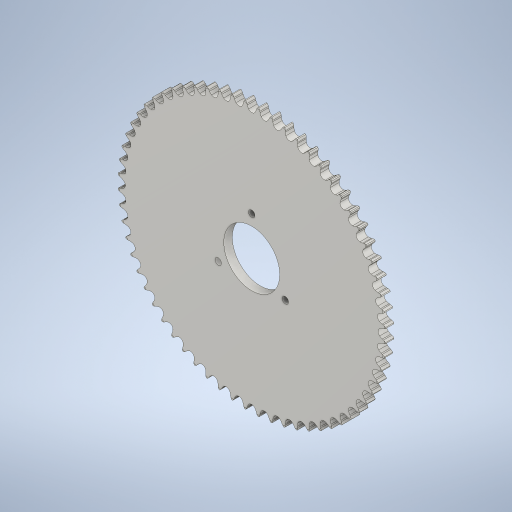
# Autodesk Inventor part: Roller Chain Sprocket2
Saved by Autodesk Inventor 2023 (Build 270158000, 158)
## iProperties
CustomPartVersion: 1
Created: 2023-09-03
Part Number: Roller Chain Sprocket2
Material: Steel
Document SubType Name: Modeling
Designer: sigit
Density: 1 g/cm^3
Appearance: Steel
Author: sigit
Autodesk Inventor part; units mm, degrees
ref_plane "YZ Plane" through (0, 0, 0) normal (1, 0, 0) x (0, 1, 0)
ref_plane "XZ Plane" through (0, 0, 0) normal (0, 1, 0) x (-1, 0, 0)
sketch "Theoretical Tooth Profile" plane through (0, 0, 0) normal (0, 0, 1) x (1, 0, 0)
  circle A0 centre (0, 0) radius 81.5201 construction
  line L0 (0, 0) -> (0, 81.5201) construction
  line L1 (0, 0) -> (7.9904, 81.1275) construction
  circle A1 centre (0, 0) radius 83.8219
  arc A2 (-1.9503, 80.1063) -> (1.9503, 80.1063) centre (0, 81.5201) ccw
  line L2 (0, 81.5201) -> (7.9904, 81.1275) construction
  line L3 (0, 81.5201) -> (3.0897, 83.7597) construction
  line L4 (3.0897, 83.7597) -> (-2.8027, 81.7523) construction
  arc A3 (3.7916, 83.7361) -> (3.0339, 82.4311) centre (6.67, 81.1924) ccw
  arc A4 (-3.0339, 82.4311) -> (-3.7916, 83.7361) centre (-6.67, 81.1924) ccw
  line L5 (-6.67, 81.1924) -> (-3.0339, 82.4311) construction
  arc A5 (-2.8027, 81.7523) -> (-1.9503, 80.1063) centre (3.0897, 83.7597) ccw
  line L6 (-2.8027, 81.7523) -> (-3.0339, 82.4311)
  arc A6 (1.9503, 80.1063) -> (2.8027, 81.7523) centre (-3.0897, 83.7597) ccw
  line L7 (3.0339, 82.4311) -> (2.8027, 81.7523)
  line L8 (0, 0) -> (4.1129, 83.7209) construction
  point P0 (3.9952, 81.3238)
  dimension "d0" = 163.0401
  dimension "d2" = 5.625
  dimension "d3" = 2.4089
  dimension "d10" = 125.938
  dimension "d11" = 17.125
  dimension "d12" = 3.816
  dimension "d13" = 6.2248
  dimension "d14" = 6.678
  dimension "d23" = 2.4
  constraints: 18 end point, 15 point on circle, 7 centre point, 3 coincident, 3 point on line, 3 symmetric about line, 3 tangent, 1 equal radius, 1 midpoint, 1 parallel, 1 vertical, 1 other
  measures "d0" diameter of A0
  measures "d2" angle of L1 L0
  measures "d3" radius of A2
  measures "d10" angle of L3 L0
  measures "d11" angle of L4 L3
  measures "d12" distance of L2.start L3.end
  measures "d13" distance of L3.end L4.end
  measures "d14" distance of A3.centre L0.end
  measures "d23" distance from line of L8.end L2
sketch "Tooth Profile" plane through (0, 0, 0) normal (0, 0, 1) x (1, 0, 0)
  arc A0 (-2.2533, 80.6685) -> (2.2533, 80.6685) centre (0, 81.5201) ccw
  arc A1 (3.5749, 83.7456) -> (2.2533, 80.6685) centre (37.5921, 67.3128) ccw
  arc A2 (-2.2533, 80.6685) -> (-3.5749, 83.7456) centre (-37.5921, 67.3128) ccw
  line L0 (0, 0) -> (0, 81.5201) construction
  line L1 (0, 81.5201) -> (2.2533, 80.6685) construction
  line L2 (0, 81.5201) -> (-2.2533, 80.6685) construction
  circle A3 centre (0, 0) radius 83.8219 projected
  dimension "d44" = 138.594
  dimension "d45" = 37.7784
  dimension "d46" = 2.4089
  constraints: 9 point on circle, 6 end point, 3 centre point, 2 tangent, 1 coincident, 1 equal radius, 1 vertical, 1 other
  measures "d44" angle of L2 L1
  measures "d45" radius of A1
  measures "d46" radius of A0
sketch "Section Profile" plane through (0, 0, 0) normal (1, 0, 0) x (0, 1, 0)
  line L0 (83.8219, 0) -> (-83.8219, 0) projected
  line L1 (73.3499, 2.6598) -> (-73.3499, 2.6598)
  line L2 (-73.3499, 2.6598) -> (-73.3499, -2.6598)
  line L3 (-73.3499, -2.6598) -> (73.3499, -2.6598)
  line L4 (73.3499, -2.6598) -> (73.3499, 2.6598)
  line L5 (73.3499, 2.6598) -> (83.8219, 2.6598) construction
  line L6 (83.8219, 2.6598) -> (83.8219, -2.6598) construction
  line L7 (83.8219, -2.6598) -> (73.3499, -2.6598) construction
  line L8 (73.3499, -2.6598) -> (73.3499, 2.6598)
  arc A0 (83.8219, 2.6118) -> (82.9468, 2.6598) centre (82.9468, -5.3402) ccw
  arc A1 (82.9468, -2.6598) -> (83.8219, -2.6118) centre (82.9468, 5.3402) ccw
  line L9 (82.9468, 2.6598) -> (0, 2.6598)
  line L10 (0, 2.6598) -> (0, -2.6598)
  line L11 (0, -2.6598) -> (82.9468, -2.6598)
  line L12 (0, 2.6598) -> (0, -2.6598)
  line L13 (83.8219, 2.6118) -> (83.8219, -2.6118)
  point P0 (0, 0)
  point P1 (0, 0)
  dimension "d30" = 5.3196
  dimension "d31" = 146.6997
  dimension "d32" = 5.3196
  dimension "d33" = 0.048
  dimension "d34" = 8
  dimension "d43" = 2.6598
  constraints: 26 end point, 7 midpoint, 5 perpendicular, 4 parallel, 4 point on circle, 3 point on line, 3 symmetric about line, 2 centre point, 2 horizontal, 2 tangent, 1 collinear, 1 other
  measures "d30" distance between parallel lines of L7 L5
  measures "d31" distance between parallel lines of L2 L4
  measures "d32" distance between parallel lines of L3 L1
  measures "d33" distance from line of L13.start L5
  measures "d34" radius of A0
  measures "d43" distance between parallel lines of L3 L0
revolve "Shroud" add sketch "Section Profile" angle 360 about axis through (0, 0, 2.6598) along (0, 0, -1) contours L10 L3 L2 L0 | L0 L2 L1 L10
revolve "Strand" add sketch "Section Profile" angle 360 about axis through (0, 0, 2.6598) along (0, 0, -1) contours L13 A1 L11 L4 L0 | L0 L4 L9 A0 L13 | L4 L3 L10 L0 | L0 L10 L1 L4
pattern_of_one "Strand Pattern"
extrude "Theoretical Tooth" cut sketch "Theoretical Tooth Profile" along normal through all both and the other way through all contours A3 L7 A6 A2 A5 L6 A4 A1 picked at (0.4214, 81.3417)
extrude "Tooth" [suppressed]
pattern_circular "Tooth Pattern" count 64 over 360 about axis through (0, 0, -10) along (0, 0, 1) of "Theoretical Tooth"
ref_plane "Timing Plane" through (0, 81.5201, 0) normal (1, 0, 0) x (0, 1, 0)
sketch "Sketch4" plane through (0, 81.5201, 2.6598) normal (0, 0, 1) x (1, 0, 0)
  circle A0 centre (0, -81.5201) radius 17.5
  circle A1 centre (0, -57.2701) radius 2
  circle A2 centre (-21.0011, -93.6451) radius 2
  circle A3 centre (21.0011, -93.6451) radius 2
  circle A4 centre (0, -81.5201) radius 17.5
  dimension "d51" = 35
  dimension "d54" = 4
  dimension "d55" = 360
  dimension "d56" = 24.25
  dimension "d57" = 35
  constraints: 5 centre point, 2 coincident, 7 other
  measures "d51" diameter of A0
  measures "d54" diameter of A1
  measures "d56" distance of A1.centre point (0, -81.52)
  measures "d57" diameter of A4
extrude "Extrusion4" cut sketch "Sketch4" against normal through all
equation "\"d3\" = 0.5 * da_Dr + da_SC"
equation "\"d12\" = 0.8 * da_Dr"
equation "\"d13\" = 1.3 * da_Dr + da_SC"
equation "\"d14\" = 1.4 * da_Dr"
equation "\"d23\" = da_Ha"
equation "\"d44\" = da_Alfa"
equation "\"d45\" = da_Re"
equation "\"d46\" = da_Ri"
equation "\"d30\" = da_Bf"
equation "\"d31\" = da_Ds"
equation "\"d32\" = da_Bs"
equation "\"d33\" = da_Ba"
equation "\"d34\" = da_Rx"
equation "\"d40\" = da_pt"
equation "\"form_type\" = 0"
equation "\"da_p\" = 8"
equation "\"da_Dr\" = 4.77"
equation "\"da_SC\" = 0.02385"
equation "\"da_Ha\" = 2.4"
equation "\"da_pt\" = 11.6"
equation "\"da_Bf\" = 5.3196"
equation "\"da_Ba\" = 0.048"
equation "\"da_Rx\" = 8"
equation "\"da_Ra\" = 0.32"
equation "\"da_Bs\" = 5.3196"
equation "\"da_Ds\" = 146.69974"
equation "\"da_Re\" = 37.7784"
equation "\"da_Ri\" = 2.40885"
equation "\"da_Alfa\" = 138.594deg"
body "Solid1"
